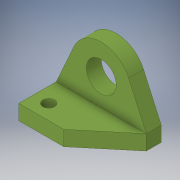
# Autodesk Inventor part: Encoder mount_right
Saved by Autodesk Inventor 2018 (Build 220112000, 112)
## iProperties
Created: 2018-03-20
Part Number: Encoder mount_right
Material: Generic
Document SubType Name: Modeling
Designer: prakh
Density: 1 g/cm^3
Appearance: Olive Green
Author: prakh
Autodesk Inventor part; units mm, degrees
ref_plane "YZ Plane" through (0, 0, 0) normal (1, 0, 0) x (0, 1, 0)
ref_plane "XZ Plane" through (0, 0, 0) normal (0, 1, 0) x (-1, 0, 0)
ref_plane "XY Plane" through (0, 0, 0) normal (0, 0, 1) x (1, 0, 0)
sketch "Sketch1" plane through (0, 0, 0) normal (0, 1, 0) x (-1, 0, 0)
  line L0 (0, 0) -> (38.1, 0)
  line L1 (38.1, 0) -> (38.1, -19.05)
  line L2 (38.1, -19.05) -> (0, -19.05)
  line L3 (0, -19.05) -> (0, 0)
  circle A0 centre (6.35, -3.175) radius 2.4765
  circle A1 centre (31.75, -3.175) radius 2.4765
  dimension "d0" = 4.953
  dimension "d1" = 4.953
  dimension "d2" = 25.4
  dimension "d3" = 6.35
  dimension "d4" = 3.175
  dimension "d5" = 6.35
  dimension "d6" = 19.05
  constraints: 8 end point, 2 centre point, 2 parallel, 1 horizontal, 1 perpendicular
  measures "d0" diameter of A0
  measures "d1" diameter of A1
  measures "d2" distance of A0.centre A1.centre
  measures "d3" distance from line of A0.centre L3
  measures "d4" distance from line of A0.centre L0
  measures "d5" distance from line of A1.centre L1
  measures "d6" distance of L2.end L0.start
extrude "Extrusion1" add sketch "Sketch1" along normal blind 6.35
sketch "Sketch2" plane through (0, 0, -19.05) normal (0, 0, -1) x (-1, 0, 0)
  line L0 (38.1, 0) -> (0, 0) projected
  line L1 (38.1, 0) -> (38.1, 6.35) projected
  line L2 (0, 6.35) -> (38.1, 6.35) projected
  line L3 (0, 0) -> (0, 6.35) projected
  circle A0 centre (19.05, 17.7546) radius 14.2748 projected
  circle A1 centre (19.05, 17.7546) radius 6.35
  line L4 (38.1, 6.35) -> (0, 6.35) projected
  line L5 (0, 6.35) -> (7.4663, 22.9612)
  line L6 (38.1, 6.35) -> (30.6337, 22.9612)
  arc A2 (30.6337, 22.9612) -> (7.4663, 22.9612) centre (19.05, 17.7546) ccw
  point P0 (0, 0)
  dimension "d9" = 6.35
  dimension "d10" = 12.7
  constraints: 4 end point, 2 centre point, 2 point on circle, 2 tangent, 1 coincident, 1 concentric
  measures "d9" radial gap between concentric circles of A2 A1
  measures "d10" diameter of A1
extrude "Extrusion2" add sketch "Sketch2" against normal blind 6.35 contours L2 A0 L6 | L5 A0 L2 | L2 A0 L5 A2 L6
sketch "Sketch3" plane through (-38.1, 0, 0) normal (0, 0, 1) x (1, 0, 0)
  line L0 (38.1, 0) -> (0, 0) projected
  line L1 (38.1, 0) -> (38.1, 6.35) projected
  line L2 (0, 6.35) -> (38.1, 6.35) projected
  line L3 (0, 0) -> (0, 6.35) projected
extrude "Extrusion3" add sketch "Sketch3" along normal blind 3.175
sketch "Sketch4" plane through (0, 6.35, 0) normal (0, 1, 0) x (1, 0, 0)
  line L0 (0, 12.7) -> (-38.1, 12.7) projected
  line L1 (-38.1, 12.7) -> (-38.1, -3.175) projected
  line L2 (0, -3.175) -> (-38.1, -3.175) projected
  line L3 (0, 12.7) -> (0, -3.175) projected
  circle A0 centre (-6.35, 3.175) radius 2.4765 projected
  circle A1 centre (-31.75, 3.175) radius 2.4765 projected
  line L4 (-38.1, -3.175) -> (0, -3.175) projected
  line L5 (0, 12.7) -> (-19.05, -3.175)
  point P0 (0, 0)
  constraints: 2 end point, 1 midpoint
extrude "Extrusion4" cut sketch "Sketch4" against normal blind 25.4 contours L3 L2 L5
equation "\"d5\" = d3"
body "Solid1"
